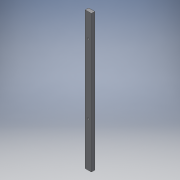
# Autodesk Inventor part: slider4a
Saved by Autodesk Inventor 2018.2 (Build 222227000, 227)
## iProperties
Created: 2018-02-09
Part Number: slider4a
Material: 一般
Document SubType Name: Modeling
Designer: SHUICHI
Density: 1 g/cm^3
Appearance: 既定
Author: SHUICHI
Autodesk Inventor part; units mm, degrees
ref_plane "YZ Plane" through (0, 0, 0) normal (1, 0, 0) x (0, 1, 0)
ref_plane "XZ Plane" through (0, 0, 0) normal (0, 1, 0) x (-1, 0, 0)
ref_plane "XY Plane" through (0, 0, 0) normal (0, 0, 1) x (1, 0, 0)
sketch "スケッチ1" plane through (0, 0, 0) normal (0, 0, 1) x (1, 0, 0)
  line L0 (0, 0) -> (11, 0)
  line L1 (11, 0) -> (11, 6)
  line L2 (11, 6) -> (0, 6)
  line L3 (0, 6) -> (0, 0)
  dimension "d0" = 11
  dimension "d1" = 6
  constraints: 8 end point, 2 parallel, 1 horizontal, 1 perpendicular
  measures "d0" distance of L2.end L1.end
  measures "d1" distance of L1.end L0.end
extrude "押し出し1" add sketch "スケッチ1" along normal blind 246
sketch "スケッチ2" plane through (0, 6, 0) normal (0, 1, 0) x (1, 0, 0)
  line L0 (11, 0) -> (0, 0) projected
  line L1 (11, -246) -> (0, -246) projected
  point P0 (5.5, -204)
  point P1 (5.5, -80)
  point P2 (5.5, 0)
  dimension "d4" = 80
  dimension "d5" = 42
  constraints: 2 vertical alignment, 1 midpoint
  measures "d4" distance from line of L0 point (5.5, -80)
  measures "d5" distance from line of L1 point (5.5, -204)
hole "穴1" at (5.5, 6, 204) at (5.5, 6, 80) direction (0, -1, 0) diameter 3 depth 8 tip angle 118
